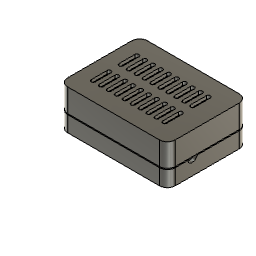
12V Analog LED Controller Enclosure (Autodesk Fusion 360 design; units mm, degrees)
Autodesk Fusion 360 part; units mm, degrees
sketch "Sketch1" plane through (0, 0, 0) normal (0, 0, 1) x (1, 0, 0) in component "PCB"
  line L0 (2, 0) -> (48, 0)
  line L1 (50, 2) -> (50, 28.5)
  line L2 (23.5, 36) -> (2, 36)
  line L3 (0, 34) -> (0, 2)
  line L4 (0, 18) -> (50, 18) construction
  circle A0 centre (18, 18) radius 1.5
  circle A1 centre (45, 18) radius 1.5
  line L5 (0, 9) -> (10.2051, 9) construction
  line L6 (0, 27) -> (10.553, 27) construction
  line L7 (25.5, 34) -> (25.5, 32.5)
  line L8 (27.5, 30.5) -> (48, 30.5)
  arc A2 (2, 36) -> (0, 34) centre (2, 34) ccw
  arc A3 (25.5, 32.5) -> (27.5, 30.5) centre (27.5, 32.5) ccw
  arc A4 (25.5, 34) -> (23.5, 36) centre (23.5, 34) ccw
  arc A5 (50, 28.5) -> (48, 30.5) centre (48, 28.5) ccw
  arc A6 (48, 0) -> (50, 2) centre (48, 2) ccw
  arc A7 (0, 2) -> (2, 0) centre (2, 2) ccw
  line L9 (41, 14) -> (30.5, 14)
  line L10 (30.5, 14) -> (30.5, 6)
  line L11 (30.5, 6) -> (41, 6)
  line L12 (41, 6) -> (41, 14)
  point P0 (50, 0)
  point P1 (0, 36)
  dimension "d1" = 50
  dimension "d2" = 36
  dimension "d3" = 3
  dimension "d4" = 3
  dimension "d5" = 18
  dimension "d6" = 45
  dimension "d7" = 30.5
  dimension "d8" = 25.5
  dimension "d9" = 9
  dimension "d10" = 27
  dimension "d11" = 2
  dimension "d88" = 10.5
  dimension "d89" = 8
  dimension "d90" = 9
  dimension "d91" = 6
  constraint horizontal L0
  constraint vertical L1
  constraint horizontal L2
  constraint vertical L3
  constraint coincident L4 A0.centre
  constraint coincident L4 A1.centre
  constraint coincident L3 L5.start
  constraint perpendicular L3 L5
  constraint coincident L3 L6.start
  constraint perpendicular L3 L6
  constraint perpendicular L2 L7
  constraint perpendicular L1 L8
  constraint coincident L1 L4.end
  constraint coincident L3 L4.start
  constraint coincident P1 L3
  constraint coincident P1 L2
  constraint tangent L3 A2
  constraint tangent L2 A2
  constraint tangent L7 A3
  constraint tangent L8 A3
  constraint equal A2 A3
  constraint tangent L2 A4
  constraint tangent L7 A4
  constraint equal A2 A4
  constraint tangent L8 A5
  constraint tangent L1 A5
  constraint equal A2 A5
  constraint coincident P0 L1
  constraint coincident P0 L0
  constraint tangent L1 A6
  constraint tangent L0 A6
  constraint equal A2 A6
  constraint coincident origin L0
  constraint coincident origin L3
  constraint tangent L0 A7
  constraint tangent L3 A7
  constraint equal A2 A7
  constraint horizontal L9
  constraint vertical L10
  constraint horizontal L11
  constraint vertical L12
  measures "d1" distance of origin P0
  measures "d2" distance of origin P1
  measures "d3" diameter of A0
  measures "d4" diameter of A1
  measures "d5" distance of L3 A0.centre
  measures "d6" distance of L3 A1.centre
  measures "d7" distance of L0 L8
  measures "d8" distance of L3 L7
  measures "d9" distance of L0 L5
  measures "d10" distance of L0 L6
  measures "d11" radius of A2
  measures "d88" distance of L9.start L9.end
  measures "d89" distance of L9.end L10.end
  measures "d90" distance of L1 L12
  measures "d91" distance of L0 L11
extrude "Extrude1" add sketch "Sketch1" along normal blind 1.4 contours L0 L1 L2 L3 L7 L8 A2 A3 A4 A5 A6 A7 | L9 L10 L11 L12 makes body 1 in component "PCB"
sketch "Sketch2" plane through (0, 0, 1.4) normal (0, 0, 1) x (-1, 0, 0) in component "PCB"
  circle A0 centre (-18, -18) radius 1.5
  circle A1 centre (-45, -18) radius 1.5
  arc A2 (-25.5, -34) -> (-23.5, -36) centre (-23.5, -34) ccw
  line L0 (-23.5, -36) -> (-2, -36)
  arc A3 (-2, -36) -> (0, -34) centre (-2, -34) ccw
  line L1 (0, -34) -> (0, -2)
  arc A4 (0, -2) -> (-2, 0) centre (-2, -2) ccw
  line L2 (-2, 0) -> (-48, 0)
  arc A5 (-48, 0) -> (-50, -2) centre (-48, -2) ccw
  line L3 (-50, -2) -> (-50, -28.5)
  arc A6 (-50, -28.5) -> (-48, -30.5) centre (-48, -28.5) ccw
  line L4 (-48, -30.5) -> (-27.5, -30.5)
  arc A7 (-25.5, -32.5) -> (-27.5, -30.5) centre (-27.5, -32.5) ccw
  line L5 (-25.5, -32.5) -> (-25.5, -34)
  line L6 (0, -9) -> (-10.2051, -9)
  line L7 (0, -27) -> (-10.553, -27)
  line L8 (0, -34.25) -> (-14, -34.25)
  line L9 (-14, -34.25) -> (-14, -19.75)
  line L10 (-14, -19.75) -> (0, -19.75)
  line L11 (0, -19.75) -> (0, -34.25)
  line L12 (0, -16.25) -> (-14, -16.25)
  line L13 (-14, -16.25) -> (-14, -1.75)
  line L14 (-14, -1.75) -> (0, -1.75)
  line L15 (0, -1.75) -> (0, -16.25)
  line L16 (-32.5, -7) -> (-43, -7)
  line L17 (-43, -7) -> (-43, -15)
  line L18 (-43, -15) -> (-32.5, -15)
  line L19 (-32.5, -15) -> (-32.5, -7)
  line L20 (-27.5, -30.5) -> (-48, -30.5)
  line L21 (-50, -2) -> (-50, -28.5)
  dimension "d14" = 14.5
  dimension "d15" = 7.25
  dimension "d16" = 14
  dimension "d17" = 7.25
  dimension "d18" = 14.5
  dimension "d92" = 10.5
  dimension "d93" = 8
  dimension "d95" = 7
  dimension "d96" = 7
  constraint horizontal L8
  constraint vertical L9
  constraint horizontal L10
  constraint vertical L11
  constraint coincident L1 L8.start
  constraint horizontal L12
  constraint vertical L13
  constraint horizontal L14
  constraint vertical L15
  constraint coincident L1 L12.start
  constraint collinear L9 L13
  constraint horizontal L16
  constraint vertical L17
  constraint horizontal L18
  constraint vertical L19
  measures "d14" distance of L8.end L9.end
  measures "d15" distance of L7 L8
  measures "d16" distance of L1 L9
  measures "d17" distance of L6 L14
  measures "d18" distance of L12 L14
  measures "d92" distance of L16.start L16.end
  measures "d93" distance of L16.start L18.end
  measures "d95" distance of L17 L21
  measures "d96" distance of L2 L16
extrude "Extrude2" add sketch "Sketch2" along normal blind 6.9 contours A3 L1 L8 L9 L10 L11 | L1 A4 L12 L13 L14 L15 bodies 1 in component "PCB"
sketch "Sketch1 (2)" plane through (0, 0, 0) normal (0, 0, 1) x (1, 0, 0) in component "Bottom"
  line L0 (1.5, 36.5) -> (48.5, 36.5)
  line L1 (50.5, 34.5) -> (50.5, 1.5)
  line L2 (48.5, -0.5) -> (1.5, -0.5)
  line L3 (-0.5, 1.5) -> (-0.5, 34.5)
  line L4 (2, 0) -> (48, 0)
  line L5 (50, 2) -> (50, 28.5)
  line L6 (0, 16.25) -> (0, 2)
  line L7 (23.5, 36) -> (2, 36)
  line L8 (49, 1) -> (1, 1)
  line L9 (1, 1) -> (1, 35)
  line L10 (1, 35) -> (49, 35)
  line L11 (49, 35) -> (49, 1)
  circle A0 centre (18, 18) radius 3
  circle A1 centre (45, 18) radius 3
  line L12 (48.1, -2.1) -> (1.9, -2.1)
  line L13 (-2.1, 1.9) -> (-2.1, 34.1)
  line L14 (1.9, 38.1) -> (48.1, 38.1)
  line L15 (52.1, 34.1) -> (52.1, 1.9)
  arc A2 (1.5, 36.5) -> (-0.5, 34.5) centre (1.5, 34.5) ccw
  arc A3 (50.5, 34.5) -> (48.5, 36.5) centre (48.5, 34.5) ccw
  arc A4 (48.5, -0.5) -> (50.5, 1.5) centre (48.5, 1.5) ccw
  arc A5 (-0.5, 1.5) -> (1.5, -0.5) centre (1.5, 1.5) ccw
  arc A6 (1.9, 38.1) -> (-2.1, 34.1) centre (1.9, 34.1) ccw
  arc A7 (52.1, 34.1) -> (48.1, 38.1) centre (48.1, 34.1) ccw
  arc A8 (48.1, -2.1) -> (52.1, 1.9) centre (48.1, 1.9) ccw
  arc A9 (-2.1, 1.9) -> (1.9, -2.1) centre (1.9, 1.9) ccw
  circle A10 centre (18, 18) radius 1.3
  circle A11 centre (45, 18) radius 1.3
  circle A12 centre (45, 18) radius 2.25
  circle A13 centre (18, 18) radius 2.1591
  point P0 (18, 18)
  point P1 (45, 18)
  dimension "d21" = 0.5
  dimension "d22" = 0.5
  dimension "d23" = 0.5
  dimension "d24" = 0.5
  dimension "d26" = 6
  dimension "d27" = 6
  dimension "d29" = 2
  dimension "d30" = 2
  dimension "d31" = 4
  dimension "d39" = 2.6
  dimension "d40" = 2.6
  dimension "d55" = 4.5
  constraint horizontal L0
  constraint vertical L1
  constraint horizontal L2
  constraint vertical L3
  constraint coincident P0 A0.centre
  constraint coincident P1 A1.centre
  constraint tangent L3 A2
  constraint tangent L0 A2
  constraint tangent L0 A3
  constraint tangent L1 A3
  constraint tangent L1 A4
  constraint tangent L2 A4
  constraint equal A3 A4
  constraint tangent L2 A5
  constraint tangent L3 A5
  constraint equal A3 A5
  constraint tangent L13 A6
  constraint tangent L14 A6
  constraint tangent L14 A7
  constraint tangent L15 A7
  constraint equal A6 A7
  constraint tangent L15 A8
  constraint tangent L12 A8
  constraint equal A6 A8
  constraint tangent L12 A9
  constraint tangent L13 A9
  constraint equal A6 A9
  constraint concentric A0 A10
  constraint concentric A10 A13
  measures "d21" distance of L2 L4
  measures "d22" distance of L1 L5
  measures "d23" distance of L3 L6
  measures "d24" distance of L0 L7
  measures "d26" diameter of A0
  measures "d27" diameter of A1
  measures "d29" radius of A2
  measures "d30" radius of A3
  measures "d31" radius of A6
  measures "d39" diameter of A10
  measures "d40" diameter of A11
  measures "d55" diameter of A12
extrude "Extrude1'" add sketch "Sketch1 (2)" against normal blind 1.4 from surface at -3 separate body contours L0 L1 L2 L3 A2 A3 A4 A5 | L8 L9 L10 L11 | A0 | A1 | L12 L13 L14 L15 A6 A7 A8 A9 | A10 | A11 | A12 | A13 makes body 2 in component "Bottom"
extrude "Extrude2'" add sketch "Sketch1 (2)" against normal up to surface (3 mm away) contours L0 L1 L2 L3 A2 A3 A4 A5 | A0 | A1 | L12 L13 L14 L15 A6 A7 A8 A9 | A10 | A11 | A12 | A13 bodies 2 in component "Bottom"
extrude "Extrude3" add sketch "Sketch1 (2)" along normal blind 4 contours L12 L13 L14 L15 A6 A7 A8 A9 bodies 2 in component "Bottom"
extrude "Extrude4" add sketch "Sketch1 (2)" along normal blind 3 contours A10 | A11 bodies 2 in component "Bottom"
chamfer "Chamfer1" distance 0.5 angle 45 8 edges at (25, 38.1, 4) (-0.9284, 36.9284, 4) (-2.1, 18, 4) (-0.9284, -0.9284, 4) (25, -2.1, 4) (50.9284, -0.9284, 4) (52.1, 18, 4) (50.9284, 36.9284, 4) on bodies 2 in component "Bottom"
sketch "Sketch1 (3)" plane through (0, 0, 4) normal (0, 0, 1) x (-1, 0, 0) in component "Top"
  arc A0 (-1.5, -36.5) -> (0.5, -34.5) centre (-1.5, -34.5) ccw
  line L0 (-1.5, -36.5) -> (-48.5, -36.5)
  arc A1 (-50.5, -34.5) -> (-48.5, -36.5) centre (-48.5, -34.5) ccw
  line L1 (-50.5, -34.5) -> (-50.5, -1.5)
  arc A2 (-48.5, 0.5) -> (-50.5, -1.5) centre (-48.5, -1.5) ccw
  line L2 (-48.5, 0.5) -> (-1.5, 0.5)
  arc A3 (0.5, -1.5) -> (-1.5, 0.5) centre (-1.5, -1.5) ccw
  line L3 (0.5, -1.5) -> (0.5, -34.5)
  line L4 (-48.1, -37.6) -> (-1.9, -37.6)
  arc A4 (-1.9, -37.6) -> (1.6, -34.1) centre (-1.9, -34.1) ccw
  line L5 (1.6, -34.1) -> (1.6, -1.9)
  arc A5 (1.6, -1.9) -> (-1.9, 1.6) centre (-1.9, -1.9) ccw
  line L6 (-1.9, 1.6) -> (-48.1, 1.6)
  arc A6 (-48.1, 1.6) -> (-51.6, -1.9) centre (-48.1, -1.9) ccw
  line L7 (-51.6, -1.9) -> (-51.6, -34.1)
  arc A7 (-51.6, -34.1) -> (-48.1, -37.6) centre (-48.1, -34.1) ccw
  circle A8 centre (-18, -18) radius 3
  circle A9 centre (-45, -18) radius 3
  arc A10 (-52.1, -34.1) -> (-48.1, -38.1) centre (-48.1, -34.1) ccw
  line L8 (-1.9, -38.1) -> (-48.1, -38.1)
  line L9 (-52.1, -34.1) -> (-52.1, -1.9)
  arc A11 (-50.5, -34.5) -> (-48.5, -36.5) centre (-48.5, -34.5) ccw
  line L10 (-1.5, -36.5) -> (-48.5, -36.5)
  arc A12 (-1.9, -38.1) -> (2.1, -34.1) centre (-1.9, -34.1) ccw
  arc A13 (-1.5, -36.5) -> (0.5, -34.5) centre (-1.5, -34.5) ccw
  line L11 (0.5, -1.5) -> (0.5, -34.5)
  line L12 (2.1, -1.9) -> (2.1, -34.1)
  arc A14 (2.1, -1.9) -> (-1.9, 2.1) centre (-1.9, -1.9) ccw
  line L13 (-48.1, 2.1) -> (-1.9, 2.1)
  line L14 (-48.5, 0.5) -> (-1.5, 0.5)
  arc A15 (0.5, -1.5) -> (-1.5, 0.5) centre (-1.5, -1.5) ccw
  arc A16 (-48.5, 0.5) -> (-50.5, -1.5) centre (-48.5, -1.5) ccw
  arc A17 (-48.1, 2.1) -> (-52.1, -1.9) centre (-48.1, -1.9) ccw
  line L15 (-50.5, -34.5) -> (-50.5, -1.5)
  circle A18 centre (-18, -18) radius 1.5
  circle A19 centre (-45, -18) radius 1.5
  dimension "d49" = 3
  dimension "d50" = 3
  measures "d49" diameter of A18
  measures "d50" diameter of A19
extrude "Extrude1''" add sketch "Sketch1 (3)" along normal blind 10 separate body contours L4 A4 L5 A5 L6 A6 L7 A7 | A10 L8 L9 A12 L12 A14 L13 A17 makes body 3 in component "Top"
extrude "Extrude2''" add sketch "Sketch1 (3)" along normal blind 1.6 from surface at 10 contours A0 L0 A1 L1 A2 L2 A3 L3 A11 L10 A13 L11 L14 A15 A16 L15 | L4 A4 L5 A5 L6 A6 L7 A7 | A8 | A9 | A10 L8 L9 A12 L12 A14 L13 A17 | A18 | A19 bodies 3 in component "Top"
extrude "Extrude3'" add sketch "Sketch1 (3)" along normal up to surface (10 mm away) and the other way up to surface (2.6 mm away) contours A8 | A9 bodies 3 in component "Top"
sketch "Sketch2 (2)" plane through (-2.1, 0, 0) normal (-1, 0, 0) x (0, -1, 0) in component "Bottom"
  line L0 (-1.9, 3.5) -> (-34.1, 3.5)
  line L1 (-34.1, 3.5) -> (-34.1, -4.4)
  line L2 (-34.1, -4.4) -> (-1.9, -4.4)
  line L3 (-1.9, -4.4) -> (-1.9, 3.5)
  line L4 (-34, 8.3) -> (-19.75, 8.3)
  line L5 (-34, 0) -> (-34, 8.3)
  line L6 (-19.75, 1.4) -> (-19.75, 8.3)
  line L7 (-16.25, 1.4) -> (-16.25, 8.3)
  line L8 (-16.25, 8.3) -> (-2, 8.3)
  line L9 (-1.75, 1.4) -> (-1.75, 8.3)
  line L10 (-34.25, 1.4) -> (-34.25, 8.3)
  line L11 (-34, 8.3) -> (-34.25, 8.3)
  line L12 (-1.75, 8.3) -> (-2, 8.3)
  line L13 (-34.25, 2.4) -> (-1.75, 2.4)
  line L14 (-18, 2.4) -> (-18, 10.9103) construction
  line L15 (-24.5, 2.4) -> (-24.5, 10.7029) construction
  line L16 (-29.15, 2.4) -> (-29.15, 13.6)
  line L17 (-29.15, 13.6) -> (-19.85, 13.6)
  line L18 (-19.85, 13.6) -> (-19.85, 2.4)
  line L19 (-1.9, 4) -> (-34.1, 4)
  line L20 (-6.85, 2.4) -> (-6.85, 13.6)
  line L21 (-16.15, 13.6) -> (-16.15, 2.4)
  line L22 (-6.85, 13.6) -> (-16.15, 13.6)
  dimension "d101" = 6.5
  dimension "d102" = 9.3
  dimension "d103" = 11.2
  dimension "d104" = 1.6
  constraint coincident L10 L13.start
  constraint coincident L9 L13.end
  constraint perpendicular L9 L13
  constraint midpoint L13 L14.start
  constraint perpendicular L13 L14
  constraint coincident L13 L15.start
  constraint perpendicular L13 L15
  constraint coincident L13 L16.start
  constraint perpendicular L4 L16
  constraint perpendicular L16 L17
  constraint coincident L13 L18.end
  constraint perpendicular L13 L18
  constraint symmetric L15 L16 L18
  constraint symmetric L14 L16.start L20.start
  constraint symmetric L14 L16.end L20.end
  constraint symmetric L14 L17.end L21.start
  constraint symmetric L14 L18.end L21.end
  measures "d101" distance of L14 L15
  measures "d102" distance of L16.end L17.end
  measures "d103" distance of L16.start L16.end
  measures "d104" distance of L13 L19
extrude "Extrude7" cut sketch "Sketch2 (2)" against normal up to surface (1.6 mm away) contours L0 L13 L20 L21 | L0 L19 L20 L21 | L8 L19 L20 L21 | L8 L20 L21 L22 | L0 L13 L16 L18 | L0 L16 L18 L19 | L4 L16 L18 L19 | L4 L16 L17 L18 bodies 3 in component "Top"
extrude "Extrude8" cut sketch "Sketch2 (2)" against normal up to surface (1.6 mm away) contours L0 L13 L20 L21 | L0 L19 L20 L21 | L0 L13 L16 L18 | L0 L16 L18 L19 bodies 2 in component "Bottom"
sketch "Sketch3" plane through (0, 0, 0) normal (1, 0, 0) x (0, 1, 0) in component "Bottom"
  line L0 (34.5, 4) -> (1.5, 4)
  line L1 (-0.5, 0) -> (-0.5, 4)
  line L2 (36.5, 0) -> (36.5, 4)
  line L3 (36.5, 4) -> (35.7929, 3.2929)
  line L4 (36.5, 4) -> (37.5, 4) construction
  line L5 (35.7929, 3.2929) -> (36.5, 2.5858)
  line L6 (35.7929, 3.2929) -> (36.7929, 3.2929) construction
  line L7 (36.5, 4) -> (36.5, 2.5858)
  line L8 (18, 4) -> (18, 7.4158) construction
  line L9 (0.2071, 3.2929) -> (-0.5, 2.5858)
  line L10 (-0.5, 4) -> (0.2071, 3.2929)
  line L11 (-0.5, 4) -> (-0.5, 2.5858)
  dimension "d60" = 135
  dimension "d61" = 1
  dimension "d62" = 45
  constraint horizontal L4
  constraint coincident L2.end L3.start
  constraint horizontal L6
  constraint coincident L2 L5.end
  constraint midpoint L0 L8.start
  constraint perpendicular L0 L8
  constraint symmetric L2.end L8 L1.end
  constraint symmetric L3.end L8 L9.start
  constraint symmetric L5.end L8 L9.end
  measures "d60" angle of L3 L4
  measures "d61" distance of L2.end L3.end
  measures "d62" angle of L5 L6
extrude "Extrude6" add sketch "Sketch3" along normal blind 40 from surface at 5 bodies 2 in component "Bottom"
sketch "Sketch3 (2)" plane through (0, 0, 0) normal (1, 0, 0) x (0, 1, 0) in component "Top"
  line L0 (35.7929, 3.2929) -> (36.5, 2.5858)
  line L1 (36.5, 4) -> (35.7929, 3.2929)
  line L2 (4.375, 4) -> (4.375, 11.7477) construction
  line L3 (36.5, 4) -> (36.5, 14) construction
  line L4 (-0.5, 4) -> (-0.5, 14) construction
  line L5 (30.2015, -0.6015) -> (34.0958, 3.2929)
  line L6 (34.0958, 3.2929) -> (29.1686, 8.2202)
  line L7 (30.1706, 8.2202) -> (29.1686, 8.2202)
  line L8 (30.2015, -0.6015) -> (36.5, 5.6971)
  line L9 (36.5, 4.2121) -> (36.5, 5.6971)
  line L10 (36.5, 4.2121) -> (35.5808, 3.2929)
  line L11 (35.5808, 3.2929) -> (30.3121, 8.5616)
  arc A0 (30.1706, 8.2202) -> (30.3121, 8.5616) centre (30.1706, 8.4202) ccw
  line L12 (-27.75, 4.2121) -> (-27.75, 5.6971)
  line L13 (-21.4515, -0.6015) -> (-25.3458, 3.2929)
  arc A1 (-21.5621, 8.5616) -> (-21.4206, 8.2202) centre (-21.4206, 8.4202) ccw
  line L14 (-27.75, 4.2121) -> (-26.8308, 3.2929)
  line L15 (-26.8308, 3.2929) -> (-21.5621, 8.5616)
  line L16 (-25.3458, 3.2929) -> (-20.4186, 8.2202)
  line L17 (-21.4515, -0.6015) -> (-27.75, 5.6971)
  line L18 (-21.4206, 8.2202) -> (-20.4186, 8.2202)
  line L19 (-27.0429, 3.2929) -> (-27.75, 2.5858)
  line L20 (-27.75, 4) -> (-27.0429, 3.2929)
  line L21 (16.15, 4) -> (19.85, 4)
  line L22 (29.15, 4) -> (34.1, 4)
  line L23 (1.9, 4) -> (6.85, 4)
  point P0 (-27.75, 4)
  dimension "d85" = 0.15
  dimension "d86" = 0.15
  dimension "d87" = 0.2
  constraint horizontal L7
  constraint coincident L3 L8.end
  constraint parallel L5 L8
  constraint coincident L3 L9.start
  constraint parallel L1 L10
  constraint parallel L0 L11
  constraint tangent L11 A0
  constraint tangent L7 A0
  constraint symmetric L0.start L2 L19.start
  constraint symmetric L0.end L2 L19.end
  constraint symmetric L1.start L2 P0
  constraint symmetric L2 L1.start P0
  constraint symmetric L2 L5.start L13.start
  constraint symmetric L2 L5.end L13.end
  constraint symmetric L2 L8.end L12.end
  constraint symmetric L2 L6.end L16.end
  constraint symmetric L2 L9.start L12.start
  constraint symmetric L2 L10.end L14.end
  constraint symmetric L2 L11.end A1.start
  constraint symmetric L2 L7.start A1.end
  constraint symmetric L2 A0 A1
  measures "d85" distance of L1 L10
  measures "d86" distance of L0 L11
  measures "d87" radius of A0
extrude "Extrude5" add sketch "Sketch3 (2)" along normal blind 40 from surface at 5 contours L8 L9 L10 L11 | L12 L14 L15 L17 bodies 3 makes body 4 at (18.3333, -26.6422, 4.5893) in component "Top"
sketch "Sketch4" plane through (52.1, 0, 0) normal (1, 0, 0) x (0, 1, 0) in component "Bottom"
  line L0 (34.1, 3.5) -> (1.9, 3.5)
  line L1 (1.9, 3.5) -> (1.9, -4.4)
  line L2 (1.9, -4.4) -> (34.1, -4.4)
  line L3 (34.1, -4.4) -> (34.1, 3.5)
  line L4 (2, 1.4) -> (28.5, 1.4)
  line L5 (34.5, 4) -> (1.5, 4)
  circle A0 centre (10.4411, 4) radius 2.5
  dimension "d72" = 5
  constraint coincident L5 A0.centre
  measures "d72" diameter of A0
extrude "Extrude7'" cut sketch "Sketch4" against normal up to surface (1.6 mm away) contours L0 A0 | L0 L5 A0 bodies 2 in component "Bottom"
sketch "Sketch5" plane through (0, 0, 0) normal (1, 0, 0) x (0, 1, 0) in component "Top"
sketch "Sketch4 (2)" plane through (0, 0, 15.6) normal (0, 0, 1) x (-1, 0, 0) in component "Top"
  line L0 (2.1, -18) -> (-52.1, -18) construction
  line L1 (-5.649, -30) -> (-52.1, -30) construction
  line L2 (-4.649, -30) -> (-5.649, -30)
  line L3 (-6.649, -29) -> (-6.649, -21)
  line L4 (-4.649, -21) -> (-4.649, -29)
  arc A0 (-5.649, -30) -> (-4.649, -29) centre (-5.649, -29) ccw
  arc A1 (-6.649, -29) -> (-5.649, -30) centre (-5.649, -29) ccw
  arc A2 (-5.649, -20) -> (-6.649, -21) centre (-5.649, -21) ccw
  arc A3 (-4.649, -21) -> (-5.649, -20) centre (-5.649, -21) ccw
  line L5 (-8.649, -21) -> (-8.649, -29)
  arc A4 (-9.649, -30) -> (-8.649, -29) centre (-9.649, -29) ccw
  line L6 (-10.649, -29) -> (-10.649, -21)
  arc A5 (-10.649, -29) -> (-9.649, -30) centre (-9.649, -29) ccw
  arc A6 (-9.649, -20) -> (-10.649, -21) centre (-9.649, -21) ccw
  arc A7 (-8.649, -21) -> (-9.649, -20) centre (-9.649, -21) ccw
  line L7 (-12.649, -21) -> (-12.649, -29)
  arc A8 (-13.649, -30) -> (-12.649, -29) centre (-13.649, -29) ccw
  line L8 (-14.649, -29) -> (-14.649, -21)
  arc A9 (-14.649, -29) -> (-13.649, -30) centre (-13.649, -29) ccw
  arc A10 (-13.649, -20) -> (-14.649, -21) centre (-13.649, -21) ccw
  arc A11 (-12.649, -21) -> (-13.649, -20) centre (-13.649, -21) ccw
  line L9 (-16.649, -21) -> (-16.649, -29)
  arc A12 (-17.649, -30) -> (-16.649, -29) centre (-17.649, -29) ccw
  line L10 (-18.649, -29) -> (-18.649, -21)
  arc A13 (-18.649, -29) -> (-17.649, -30) centre (-17.649, -29) ccw
  arc A14 (-17.649, -20) -> (-18.649, -21) centre (-17.649, -21) ccw
  arc A15 (-16.649, -21) -> (-17.649, -20) centre (-17.649, -21) ccw
  line L11 (-20.649, -21) -> (-20.649, -29)
  arc A16 (-21.649, -30) -> (-20.649, -29) centre (-21.649, -29) ccw
  line L12 (-22.649, -29) -> (-22.649, -21)
  arc A17 (-22.649, -29) -> (-21.649, -30) centre (-21.649, -29) ccw
  arc A18 (-21.649, -20) -> (-22.649, -21) centre (-21.649, -21) ccw
  arc A19 (-20.649, -21) -> (-21.649, -20) centre (-21.649, -21) ccw
  line L13 (-24.649, -21) -> (-24.649, -29)
  arc A20 (-25.649, -30) -> (-24.649, -29) centre (-25.649, -29) ccw
  line L14 (-26.649, -29) -> (-26.649, -21)
  arc A21 (-26.649, -29) -> (-25.649, -30) centre (-25.649, -29) ccw
  arc A22 (-25.649, -20) -> (-26.649, -21) centre (-25.649, -21) ccw
  arc A23 (-24.649, -21) -> (-25.649, -20) centre (-25.649, -21) ccw
  line L15 (-28.649, -21) -> (-28.649, -29)
  arc A24 (-29.649, -30) -> (-28.649, -29) centre (-29.649, -29) ccw
  line L16 (-30.649, -29) -> (-30.649, -21)
  arc A25 (-30.649, -29) -> (-29.649, -30) centre (-29.649, -29) ccw
  arc A26 (-29.649, -20) -> (-30.649, -21) centre (-29.649, -21) ccw
  arc A27 (-28.649, -21) -> (-29.649, -20) centre (-29.649, -21) ccw
  line L17 (-32.649, -21) -> (-32.649, -29)
  arc A28 (-33.649, -30) -> (-32.649, -29) centre (-33.649, -29) ccw
  line L18 (-34.649, -29) -> (-34.649, -21)
  arc A29 (-34.649, -29) -> (-33.649, -30) centre (-33.649, -29) ccw
  arc A30 (-33.649, -20) -> (-34.649, -21) centre (-33.649, -21) ccw
  arc A31 (-32.649, -21) -> (-33.649, -20) centre (-33.649, -21) ccw
  line L19 (-36.649, -21) -> (-36.649, -29)
  arc A32 (-37.649, -30) -> (-36.649, -29) centre (-37.649, -29) ccw
  line L20 (-38.649, -29) -> (-38.649, -21)
  arc A33 (-38.649, -29) -> (-37.649, -30) centre (-37.649, -29) ccw
  arc A34 (-37.649, -20) -> (-38.649, -21) centre (-37.649, -21) ccw
  arc A35 (-36.649, -21) -> (-37.649, -20) centre (-37.649, -21) ccw
  line L21 (-40.649, -21) -> (-40.649, -29)
  arc A36 (-41.649, -30) -> (-40.649, -29) centre (-41.649, -29) ccw
  line L22 (-42.649, -29) -> (-42.649, -21)
  arc A37 (-42.649, -29) -> (-41.649, -30) centre (-41.649, -29) ccw
  arc A38 (-41.649, -20) -> (-42.649, -21) centre (-41.649, -21) ccw
  arc A39 (-40.649, -21) -> (-41.649, -20) centre (-41.649, -21) ccw
  line L23 (-26.649, -7) -> (-26.649, -15)
  line L24 (-32.649, -15) -> (-32.649, -7)
  arc A40 (-9.649, -6) -> (-10.649, -7) centre (-9.649, -7) ccw
  line L25 (-16.649, -15) -> (-16.649, -7)
  arc A41 (-26.649, -15) -> (-25.649, -16) centre (-25.649, -15) ccw
  arc A42 (-17.649, -16) -> (-16.649, -15) centre (-17.649, -15) ccw
  arc A43 (-12.649, -7) -> (-13.649, -6) centre (-13.649, -7) ccw
  arc A44 (-9.649, -16) -> (-8.649, -15) centre (-9.649, -15) ccw
  arc A45 (-5.649, -6) -> (-6.649, -7) centre (-5.649, -7) ccw
  arc A46 (-17.649, -6) -> (-18.649, -7) centre (-17.649, -7) ccw
  arc A47 (-16.649, -7) -> (-17.649, -6) centre (-17.649, -7) ccw
  line L26 (-24.649, -15) -> (-24.649, -7)
  arc A48 (-38.649, -15) -> (-37.649, -16) centre (-37.649, -15) ccw
  arc A49 (-21.649, -6) -> (-22.649, -7) centre (-21.649, -7) ccw
  line L27 (-38.649, -7) -> (-38.649, -15)
  arc A50 (-21.649, -16) -> (-20.649, -15) centre (-21.649, -15) ccw
  line L28 (-18.649, -7) -> (-18.649, -15)
  arc A51 (-36.649, -7) -> (-37.649, -6) centre (-37.649, -7) ccw
  arc A52 (-4.649, -7) -> (-5.649, -6) centre (-5.649, -7) ccw
  line L29 (-10.649, -7) -> (-10.649, -15)
  arc A53 (-25.649, -6) -> (-26.649, -7) centre (-25.649, -7) ccw
  arc A54 (-42.649, -15) -> (-41.649, -16) centre (-41.649, -15) ccw
  arc A55 (-10.649, -15) -> (-9.649, -16) centre (-9.649, -15) ccw
  arc A56 (-28.649, -7) -> (-29.649, -6) centre (-29.649, -7) ccw
  line L30 (-36.649, -15) -> (-36.649, -7)
  line L31 (-6.649, -7) -> (-6.649, -15)
  arc A57 (-33.649, -6) -> (-34.649, -7) centre (-33.649, -7) ccw
  arc A58 (-41.649, -16) -> (-40.649, -15) centre (-41.649, -15) ccw
  arc A59 (-30.649, -15) -> (-29.649, -16) centre (-29.649, -15) ccw
  line L32 (-40.649, -15) -> (-40.649, -7)
  arc A60 (-8.649, -7) -> (-9.649, -6) centre (-9.649, -7) ccw
  line L33 (-42.649, -7) -> (-42.649, -15)
  arc A61 (-5.649, -16) -> (-4.649, -15) centre (-5.649, -15) ccw
  line L34 (-20.649, -15) -> (-20.649, -7)
  arc A62 (-41.649, -6) -> (-42.649, -7) centre (-41.649, -7) ccw
  arc A63 (-14.649, -15) -> (-13.649, -16) centre (-13.649, -15) ccw
  arc A64 (-20.649, -7) -> (-21.649, -6) centre (-21.649, -7) ccw
  arc A65 (-24.649, -7) -> (-25.649, -6) centre (-25.649, -7) ccw
  line L35 (-4.649, -15) -> (-4.649, -7)
  arc A66 (-33.649, -16) -> (-32.649, -15) centre (-33.649, -15) ccw
  line L36 (-22.649, -7) -> (-22.649, -15)
  arc A67 (-6.649, -15) -> (-5.649, -16) centre (-5.649, -15) ccw
  arc A68 (-34.649, -15) -> (-33.649, -16) centre (-33.649, -15) ccw
  line L37 (-28.649, -15) -> (-28.649, -7)
  line L38 (-4.649, -6) -> (-5.649, -6)
  arc A69 (-25.649, -16) -> (-24.649, -15) centre (-25.649, -15) ccw
  line L39 (-14.649, -7) -> (-14.649, -15)
  arc A70 (-13.649, -16) -> (-12.649, -15) centre (-13.649, -15) ccw
  arc A71 (-32.649, -7) -> (-33.649, -6) centre (-33.649, -7) ccw
  arc A72 (-13.649, -6) -> (-14.649, -7) centre (-13.649, -7) ccw
  arc A73 (-29.649, -6) -> (-30.649, -7) centre (-29.649, -7) ccw
  line L40 (-30.649, -7) -> (-30.649, -15)
  arc A74 (-18.649, -15) -> (-17.649, -16) centre (-17.649, -15) ccw
  line L41 (-34.649, -7) -> (-34.649, -15)
  arc A75 (-29.649, -16) -> (-28.649, -15) centre (-29.649, -15) ccw
  line L42 (-12.649, -15) -> (-12.649, -7)
  arc A76 (-37.649, -6) -> (-38.649, -7) centre (-37.649, -7) ccw
  arc A77 (-40.649, -7) -> (-41.649, -6) centre (-41.649, -7) ccw
  arc A78 (-37.649, -16) -> (-36.649, -15) centre (-37.649, -15) ccw
  arc A79 (-22.649, -15) -> (-21.649, -16) centre (-21.649, -15) ccw
  line L43 (-8.649, -15) -> (-8.649, -7)
  arc A80 (2.1, -1.9) -> (-1.9, 2.1) centre (-1.9, -1.9) ccw
  line L44 (-1.9, 2.1) -> (-48.1, 2.1)
  arc A81 (-48.1, 2.1) -> (-52.1, -1.9) centre (-48.1, -1.9) ccw
  line L45 (-52.1, -1.9) -> (-52.1, -34.1)
  arc A82 (-52.1, -34.1) -> (-48.1, -38.1) centre (-48.1, -34.1) ccw
  line L46 (-48.1, -38.1) -> (-1.9, -38.1)
  arc A83 (-1.9, -38.1) -> (2.1, -34.1) centre (-1.9, -34.1) ccw
  line L47 (2.1, -34.1) -> (2.1, -1.9)
  dimension "d75" = 12
  dimension "d77" = 2
  dimension "d78" = 1
  dimension "d81" = -4
  dimension "d82" = 0
  constraint horizontal L2
  constraint vertical L3
  constraint vertical L4
  constraint coincident L1 L2.start
  constraint coincident L2.start L4
  constraint tangent L4 A0
  constraint tangent L1 A0
  constraint tangent L2 A1
  constraint tangent L3 A1
  constraint equal A0 A1
  constraint tangent L3 A2
  constraint equal A0 A2
  constraint tangent L4 A3
  constraint equal A0 A3
  constraint coincident A2.start A3.end
  constraint symmetric L0 L2.start L38.start
  constraint symmetric L0 L4.end A52.start
  constraint symmetric L0 L1.start A45.start
  constraint symmetric L0 A0 A52
  constraint symmetric L0 L3.start A45.end
  constraint symmetric L0 A1 A45
  constraint symmetric L0 L3.end L31.end
  constraint symmetric L0 A2.start A61.start
  constraint symmetric L0 A2 A67
  constraint symmetric L0 L4.start A61.end
  constraint symmetric L0 A3 A61
  constraint symmetric L0 L5.start A44.end
  constraint symmetric L0 L5.end A60.start
  constraint symmetric L0 A4.start A40.start
  constraint symmetric L0 A4 A60
  constraint symmetric L0 L6.start A40.end
  constraint symmetric L0 L6.end L29.end
  constraint symmetric L0 A5 A40
  constraint symmetric L0 A6.start A44.start
  constraint symmetric L0 A6 A55
  constraint symmetric L0 A7 A44
  constraint symmetric L0 L7.start A70.end
  constraint symmetric L0 L7.end A43.start
  constraint symmetric L0 A8.start A43.end
  constraint symmetric L0 A8 A43
  constraint symmetric L0 L8.start L39.start
  constraint symmetric L0 L8.end A63.start
  constraint symmetric L0 A9 A72
  constraint symmetric L0 A10.start A63.end
  constraint symmetric L0 A10 A63
  constraint symmetric L0 A11 A70
  constraint symmetric L0 L9.start L25.start
  constraint symmetric L0 L9.end L25.end
  constraint symmetric L0 A12.start A46.start
  constraint symmetric L0 A12 A47
  constraint symmetric L0 L10.start A46.end
  constraint symmetric L0 L10.end L28.end
  constraint symmetric L0 A13 A46
  constraint symmetric L0 A14.start A42.start
  constraint symmetric L0 A14 A74
  constraint symmetric L0 A15 A42
  constraint symmetric L0 L11.start A50.end
  constraint symmetric L0 L11.end L34.end
  constraint symmetric L0 A16.start A49.start
  constraint symmetric L0 A16 A64
  constraint symmetric L0 L12.start A49.end
  constraint symmetric L0 L12.end L36.end
  constraint symmetric L0 A17 A49
  constraint symmetric L0 A18.start A50.start
  constraint symmetric L0 A18 A79
  constraint symmetric L0 A19 A50
  constraint symmetric L0 L13.start L26.start
  constraint symmetric L0 L13.end L26.end
  constraint symmetric L0 A20.start A53.start
  constraint symmetric L0 A20 A65
  constraint symmetric L0 L14.start L23.start
  constraint symmetric L0 L14.end L23.end
  constraint symmetric L0 A21 A53
  constraint symmetric L0 A22.start A41.end
  constraint symmetric L0 A22 A41
  constraint symmetric L0 A23 A69
  constraint symmetric L0 L15.start L37.start
  constraint symmetric L0 L15.end A56.start
  constraint symmetric L0 A24.start A56.end
  constraint symmetric L0 A24 A56
  constraint symmetric L0 L16.start A73.end
  constraint symmetric L0 L16.end A59.start
  constraint symmetric L0 A25 A73
  constraint symmetric L0 A26.start A59.end
  constraint symmetric L0 A26 A59
  constraint symmetric L0 A27 A75
  constraint symmetric L0 L17.start L24.start
  constraint symmetric L0 L17.end L24.end
  constraint symmetric L0 A28.start A57.start
  constraint symmetric L0 A28 A71
  constraint symmetric L0 L18.start A57.end
  constraint symmetric L0 L18.end A68.start
  constraint symmetric L0 A29 A57
  constraint symmetric L0 A30.start A66.start
  constraint symmetric L0 A30 A68
  constraint symmetric L0 A31 A66
  constraint symmetric L0 L19.start L30.start
  constraint symmetric L0 L19.end A51.start
  constraint symmetric L0 A32.start A51.end
  constraint symmetric L0 A32 A51
  constraint symmetric L0 L20.start L27.start
  constraint symmetric L0 L20.end A48.start
  constraint symmetric L0 A33 A76
  constraint symmetric L0 A34.start A48.end
  constraint symmetric L0 A34 A48
  constraint symmetric L0 A35 A78
  constraint symmetric L0 L21.start A58.end
  constraint symmetric L0 L21.end L32.end
  constraint symmetric L0 A36.start A62.start
  constraint symmetric L0 A36 A77
  constraint symmetric L0 L22.start L33.start
  constraint symmetric L0 L22.end A54.start
  constraint symmetric L0 A37 A62
  constraint symmetric L0 A38.start A54.end
  constraint symmetric L0 A38 A54
  constraint symmetric L0 A39 A58
  measures "d75" distance of L0 L1
  measures "d77" distance of L3 L4
  measures "d78" radius of A0
extrude "Extrude6'" cut sketch "Sketch4 (2)" against normal up to surface (1.6 mm away) contours L3 L4 A0 A1 A2 A3 | L5 A4 L6 A5 A6 A7 | L7 A8 L8 A9 A10 A11 | L9 A12 L10 A13 A14 A15 | L11 A16 L12 A17 A18 A19 | L13 A20 L14 A21 A22 A23 | L15 A24 L16 A25 A26 A27 | L17 A28 L18 A29 A30 A31 | L19 A32 L20 A33 A34 A35 | L21 A36 L22 A37 A38 A39 | L23 A41 L26 A53 A65 A69 | L24 A57 A66 A68 A71 L41 | A40 A44 L29 A55 A60 L43 | L25 A42 A46 A47 L28 A74 | A43 A63 L39 A70 A72 L42 | A45 A52 L31 A61 L35 A67 | A48 L27 A51 L30 A76 A78 | A49 A50 L34 A64 L36 A79 | A54 A58 L32 L33 A62 A77 | A56 A59 L37 A73 L40 A75 bodies 3 in component "Top"
extrude "Extrude3''" add sketch "Sketch2" along normal blind 10.1 contours L16 L17 L18 L19 bodies 1 in component "PCB"
component "PCB" placed x (1, 0, 0) y (0, 1, 0) z (0, 0, 1) at (0, 0, 0)
component "Bottom" placed x (1, 0, 0) y (0, 1, 0) z (0, 0, 1) at (0, 0, 0)
component "Top" placed x (1, 0, 0) y (0, 1, 0) z (0, 0, 1) at (0, 0, 0)
equation "d15 = ( 14.5 / 2 ) * 1 mm"
named bodies: "PCB", "Bottom", "Top"
